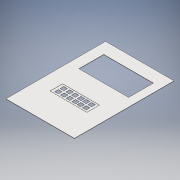
# Autodesk Inventor part: Pieza4
Saved by Autodesk Inventor 2018 (Build 220112000, 112)
## iProperties
Created: 2022-01-18
Part Number: Pieza4
Material: Plástico LCP
Document SubType Name: Chapa
Designer: stige
Density: 1.626 g/cm^3
Sheet Metal Rule: Por defecto_mm
Appearance: Suave - Blanco
Author: stige
Autodesk Inventor part; units mm, degrees
ref_plane "YZ Plane" through (0, 0, 0) normal (1, 0, 0) x (0, 1, 0)
ref_plane "XZ Plane" through (0, 0, 0) normal (0, 1, 0) x (-1, 0, 0)
ref_plane "XY Plane" through (0, 0, 0) normal (0, 0, 1) x (1, 0, 0)
sketch "Boceto1" plane through (0, 0, 0) normal (0, 0, 1) x (1, 0, 0)
  line L0 (-55, 80) -> (55, 80)
  line L1 (55, 80) -> (55, -80)
  line L2 (55, -80) -> (-55, -80)
  line L3 (-55, -80) -> (-55, 80)
  line L4 (-55, 80) -> (55, -80) construction
  line L5 (55, 80) -> (-55, -80) construction
  point P0 (0, 0)
  dimension "d0" = 110
  dimension "d1" = 160
  measures "d0" distance of L1.end L2.end
  measures "d1" distance of L0.end L1.end
extrude "Placa1" add sketch "Boceto1" along normal blind 0.5
sketch "Boceto2" plane through (0, 0, 0.5) normal (0, 0, 1) x (1, 0, 0)
  line L0 (-38.3122, 60.4154) -> (41.6878, 60.4154)
  line L1 (41.6878, 60.4154) -> (41.6878, 20.4154)
  line L2 (41.6878, 20.4154) -> (-38.3122, 20.4154)
  line L3 (-38.3122, 20.4154) -> (-38.3122, 60.4154)
  line L4 (-26.0335, -16.1653) -> (-26.0335, -22.1653)
  line L5 (-26.0335, -22.1653) -> (-20.0335, -22.1653)
  line L6 (-20.0335, -22.1653) -> (-20.0335, -16.1653)
  line L7 (-20.0335, -16.1653) -> (-26.0335, -16.1653)
  line L8 (-16.6334, -22.1653) -> (-16.6334, -16.1653)
  line L9 (-16.6334, -16.1653) -> (-10.6334, -16.1653)
  line L10 (-10.6334, -16.1653) -> (-10.6334, -22.1653)
  line L11 (-10.6334, -22.1653) -> (-16.6334, -22.1653)
  line L12 (-7.6728, -22.1653) -> (-7.6728, -16.1653)
  line L13 (-7.6728, -16.1653) -> (-1.6728, -16.1653)
  line L14 (-1.6728, -16.1653) -> (-1.6728, -22.1653)
  line L15 (-1.6728, -22.1653) -> (-7.6728, -22.1653)
  line L16 (1.6878, -22.1653) -> (1.6878, -16.1653)
  line L17 (1.6878, -16.1653) -> (7.6878, -16.1653)
  line L18 (7.6878, -16.1653) -> (7.6878, -22.1653)
  line L19 (7.6878, -22.1653) -> (1.6878, -22.1653)
  line L20 (10.0278, -16.1653) -> (10.0278, -22.1653)
  line L21 (10.0278, -22.1653) -> (16.0278, -22.1653)
  line L22 (16.0278, -22.1653) -> (16.0278, -16.1653)
  line L23 (16.0278, -16.1653) -> (10.0278, -16.1653)
  line L24 (18.758, -22.1653) -> (18.758, -16.1653)
  line L25 (18.758, -16.1653) -> (24.758, -16.1653)
  line L26 (24.758, -16.1653) -> (24.758, -22.1653)
  line L27 (24.758, -22.1653) -> (18.758, -22.1653)
  line L28 (-26.0335, -24.8985) -> (-26.0335, -30.8985)
  line L29 (-26.0335, -30.8985) -> (-20.0335, -30.8985)
  line L30 (-20.0335, -30.8985) -> (-20.0335, -24.8985)
  line L31 (-20.0335, -24.8985) -> (-26.0335, -24.8985)
  line L32 (-16.6334, -24.8985) -> (-16.6334, -30.8985)
  line L33 (-16.6334, -30.8985) -> (-10.6334, -30.8985)
  line L34 (-10.6334, -30.8985) -> (-10.6334, -24.8985)
  line L35 (-10.6334, -24.8985) -> (-16.6334, -24.8985)
  line L36 (-7.6728, -24.8985) -> (-7.6728, -30.8985)
  line L37 (-7.6728, -30.8985) -> (-1.6728, -30.8985)
  line L38 (-1.6728, -30.8985) -> (-1.6728, -24.8985)
  line L39 (-1.6728, -24.8985) -> (-7.6728, -24.8985)
  line L40 (1.6878, -24.8985) -> (1.6878, -30.8985)
  line L41 (1.6878, -30.8985) -> (7.6878, -30.8985)
  line L42 (7.6878, -30.8985) -> (7.6878, -24.8985)
  line L43 (7.6878, -24.8985) -> (1.6878, -24.8985)
  line L44 (16.0278, -24.8985) -> (16.0278, -30.8985)
  line L45 (10.0278, -30.8985) -> (10.0278, -24.8985)
  line L46 (16.0278, -24.8985) -> (10.0278, -24.8985)
  line L47 (10.0278, -30.8985) -> (16.0278, -30.8985)
  line L48 (18.758, -24.8985) -> (18.758, -30.8985)
  line L49 (18.758, -30.8985) -> (24.758, -30.8985)
  line L50 (24.758, -30.8985) -> (24.758, -24.8985)
  line L51 (24.758, -24.8985) -> (18.758, -24.8985)
  point P0 (0, 0)
  constraints: 104 end point, 35 perpendicular, 24 point on line, 7 vertical, 1 horizontal, 1 parallel
extrude "Extrusión1" cut sketch "Boceto2" against normal blind 10
sketch "Boceto3" plane through (0, 0, 0.5) normal (0, 0, 1) x (1, 0, 0)
  line L0 (-30.451, -13.5858) -> (-30.451, -33.7304)
  line L1 (-30.451, -33.7304) -> (28.8113, -33.7304)
  line L2 (28.8113, -33.7304) -> (28.8113, -13.5858)
  line L3 (28.8113, -13.5858) -> (-30.451, -13.5858)
  point P0 (0, 0)
  constraints: 8 end point, 2 perpendicular, 2 vertical
extrude "Extrusión2" cut sketch "Boceto3" against normal blind 0.2
equation "\"d2\" = Grosor"
equation "\"Radio_pliegue\" = Grosor"
equation "\"Anchura_desahogo_plegado\" = Grosor"
equation "\"Profundidad_desahogo_plegado\" = 0.5 * Grosor"
equation "\"Tamaño_destalonado\" = 4 * Grosor"
equation "\"Remanente_mínimo\" = 2 * Grosor"
equation "\"Radiodetransición\" = Radio_pliegue"
equation "\"Tamaño_de_radio_de_Jacobi\" = Radio_pliegue"
equation "\"TamañoSeparación\" = Grosor"
equation "\"Grosor\" = 0.5"
